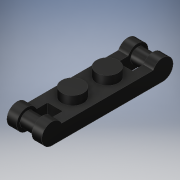
# Autodesk Inventor part: Weird circle things
Saved by Autodesk Inventor 2017 (Build 210142000, 142)
## iProperties
Created: 2018-05-11
Part Number: Weird circle things
Material: ABS Plastic
Document SubType Name: Modeling
Designer: Kyle
Density: 1.06 g/cm^3
Appearance: Glossy - Black
Author: Kyle
Autodesk Inventor part; units mm, degrees
ref_plane "YZ Plane" through (0, 0, 0) normal (1, 0, 0) x (0, 1, 0)
ref_plane "XZ Plane" through (0, 0, 0) normal (0, 1, 0) x (-1, 0, 0)
ref_plane "XY Plane" through (0, 0, 0) normal (0, 0, 1) x (1, 0, 0)
sketch "Sketch1" plane through (0, 0, 0) normal (0, 1, 0) x (-1, 0, 0)
  line L0 (0, 0) -> (7.7978, 0) construction
  line L1 (7.7978, 0) -> (7.7978, -21.1531) construction
  line L2 (7.7978, -21.1531) -> (0, -21.1531) construction
  line L3 (0, -21.1531) -> (0, 0) construction
  line L4 (7.7978, -10.5766) -> (7.7978, -2.7788) construction
  line L5 (7.7978, -2.7788) -> (0, -2.7788) construction
  line L6 (0, -2.7788) -> (0, -18.3744) construction
  line L7 (0, -18.3744) -> (7.7978, -18.3744) construction
  line L8 (7.7978, -18.3744) -> (7.7978, -2.7788) construction
  line L9 (7.7978, 0) -> (5.5905, 0) construction
  line L10 (5.5905, 0) -> (5.5905, -2.7788) construction
  line L11 (5.5905, -2.7788) -> (7.7978, -2.7788) construction
  line L12 (7.7978, -2.7788) -> (7.7978, 0) construction
  line L13 (7.7978, -10.5766) -> (0, -10.5766) construction
  line L14 (5.5905, -21.1531) -> (5.5905, -18.3744) construction
  line L15 (3.8989, 0) -> (3.8989, -21.1531) construction
  line L16 (2.2073, 0) -> (2.2073, -2.7788) construction
  line L17 (2.2073, -21.1531) -> (2.2073, -18.3744) construction
  line L18 (7.7978, 0) -> (7.7978, -21.1531)
  line L19 (7.7978, -21.1531) -> (5.5905, -21.1531)
  line L20 (5.5905, -21.1531) -> (5.5905, -18.3744)
  line L21 (5.5905, -18.3744) -> (2.2073, -18.3744)
  line L22 (2.2073, -18.3744) -> (2.2073, -21.1531)
  line L23 (2.2073, -21.1531) -> (0, -21.1531)
  line L24 (0, -21.1531) -> (0, 0)
  line L25 (0, 0) -> (2.2073, 0)
  line L26 (2.2073, 0) -> (2.2073, -2.7788)
  line L27 (2.2073, -2.7788) -> (5.5905, -2.7788)
  line L28 (5.5905, -2.7788) -> (5.5905, 0)
  line L29 (5.5905, 0) -> (7.7978, 0)
  dimension "d0" = 7.7978
  dimension "d1" = 21.1531
  dimension "d2" = 7.7978
  dimension "d3" = 7.7978
  dimension "d4" = 15.5956
  dimension "d5" = 2.2073
  constraints: 60 end point, 6 collinear, 6 parallel, 6 symmetric about line, 5 perpendicular, 4 midpoint, 3 horizontal, 2 point on line
  measures "d0" distance of L1.end L2.end
  measures "d1" distance of L0.end L1.end
  measures "d2" distance of L4.start L4.end
  measures "d3" distance of L7.end L6.end
  measures "d4" distance of L6.end L5.end
  measures "d5" distance of L11.end L10.end
extrude "Extrusion1" add sketch "Sketch1" along normal blind 3.236
sketch "Sketch2" plane through (0, 3.236, 0) normal (0, 1, 0) x (1, 0, 0)
  line L0 (0, 0) -> (0, 21.1531) construction
  line L1 (0, 10.5766) -> (-7.7978, 10.5766) construction
  line L2 (-7.7978, 21.1531) -> (-7.7978, 0) construction
  line L3 (0, 10.5766) -> (-3.8989, 10.5766) construction
  line L4 (-3.8989, 10.5766) -> (-3.8989, 6.6777) construction
  line L5 (-3.8989, 6.6777) -> (0, 6.6777) construction
  line L6 (0, 6.6777) -> (0, 10.5766) construction
  circle A0 centre (-3.8989, 6.6777) radius 2.4498
  dimension "d8" = 3.8989
  dimension "d9" = 3.8989
  dimension "d10" = 4.8997
  constraints: 10 end point, 2 midpoint, 2 parallel, 1 centre point, 1 coincident, 1 horizontal, 1 perpendicular
  measures "d8" distance of L5.end L4.end
  measures "d9" distance of L4.end L3.end
  measures "d10" diameter of A0
extrude "Extrusion2" add sketch "Sketch2" along normal blind 1.9837
pattern_linear "Rectangular Pattern1" count 2 spacing 7.7978 along (0, 0, -1) of "Extrusion2"
shell "Shell1" thickness 1.4732 removed faces 1 at (-3.335, 0, -7.9773)
sketch "Sketch3" plane through (-6.3246, 1.7628, -16.9012) normal (0, -1, 0) x (1, 0, 0)
  circle A0 centre (2.4257, 10.2235) radius 2.4498 construction
  circle A1 centre (2.4257, 2.4257) radius 2.4498 construction
  line L0 (2.4257, 10.2235) -> (2.4257, 2.4257) construction
  circle A2 centre (2.4257, 6.3246) radius 1.4491
  point P0 (6.3246, 16.9012)
  constraints: 2 end point, 1 centre point, 1 midpoint, 1 vertical
extrude "Extrusion3" add sketch "Sketch3" along normal up to surface (1.7628 mm away)
ref_plane "Work Plane1" through (0, 2.3178, 0) normal (0, -1, 0) x (1, 0, 0)
sketch "Sketch5" plane through (0, 2.3178, 0) normal (0, -1, 0) x (1, 0, 0)
  line L0 (-7.7978, -21.1531) -> (-7.7978, 0) construction
  line L1 (-7.7978, 0) -> (-7.7978, 1.8186) construction
  line L2 (-7.7978, 0) -> (-5.9792, 0) construction
  line L3 (-7.7978, 1.8186) -> (0, 1.8186) construction
  line L4 (0, 1.8186) -> (0, 4.1377) construction
  line L5 (0, 4.1377) -> (-7.7978, 4.1377) construction
  line L6 (-7.7978, 4.1377) -> (-7.7978, 1.8186) construction
  line L7 (-7.7978, 4.1377) -> (-5.5905, 4.1377) construction
  line L8 (-7.7978, 4.1377) -> (-5.5905, 4.1377) construction
  line L9 (-5.5905, 4.1377) -> (-2.2073, 4.1377) construction
  line L10 (-2.2073, 4.1377) -> (-2.2073, 3.4366) construction
  line L11 (-2.2073, 3.4366) -> (-5.5905, 3.4366) construction
  line L12 (-5.5905, 3.4366) -> (-5.5905, 4.1377) construction
  line L13 (-7.7978, 1.8186) -> (0, 1.8186)
  line L14 (0, 1.8186) -> (0, 4.1377)
  line L15 (0, 4.1377) -> (-2.2073, 4.1377)
  line L16 (-2.2073, 4.1377) -> (-2.2073, 3.4366)
  line L17 (-2.2073, 3.4366) -> (-5.5905, 3.4366)
  line L18 (-5.5905, 3.4366) -> (-5.5905, 4.1377)
  line L19 (-5.5905, 4.1377) -> (-7.7978, 4.1377)
  line L20 (-7.7978, 4.1377) -> (-7.7978, 1.8186)
  dimension "d28" = 1.8186
  dimension "d29" = 90
  dimension "d30" = 7.7978
  dimension "d31" = 2.319
  dimension "d32" = 2.2073
  dimension "d33" = 0
  dimension "d34" = 3.3833
  dimension "d35" = 0.701
  constraints: 40 end point, 6 perpendicular, 5 horizontal, 4 collinear, 4 parallel, 2 equal length, 1 vertical
  measures "d28" distance of L0.end L1.end
  measures "d29" angle of L2 L1
  measures "d30" distance of L5.end L4.end
  measures "d31" distance of L4.end L3.end
  measures "d32" distance of L5.end L7.end
  measures "d33" distance between parallel lines of L7 L8
  measures "d34" distance of L10.end L11.end
  measures "d35" distance of L9.end L10.end
revolve "Revolution1" add sketch "Sketch5" angle 360 about axis through (-7.7978, 2.3178, 1.8186) along (1, 0, 0)
sketch "Sketch6" plane through (-2.2073, 0, 0) normal (0, 0, 1) x (1, 0, 0)
  line L0 (2.2073, 0) -> (0, 0) projected
  line L1 (0, 0) -> (0, 3.236) projected
  line L2 (2.2073, 0) -> (0, 0)
  line L3 (0, 0) -> (0, 3.236)
  line L4 (0, 3.236) -> (2.2073, 3.236)
  line L5 (2.2073, 3.236) -> (2.2073, 0)
  line L6 (-3.3833, 0) -> (-5.5905, 0) projected
  line L7 (-3.3833, 0) -> (-3.3833, 3.236) projected
  line L8 (-5.5905, 0) -> (-3.3833, 0)
  line L9 (-3.3833, 0) -> (-3.3833, 3.236)
  line L10 (-3.3833, 3.236) -> (-5.5905, 3.236)
  line L11 (-5.5905, 3.236) -> (-5.5905, 0)
  constraints: 16 end point, 4 parallel, 2 horizontal, 2 perpendicular
extrude "Extrusion4" add sketch "Sketch6" along normal up to surface round surface about axis through (-1.1036, 2.3178, 1.8186) along (1, 0, 0) radius 2.319 far side no
ref_plane "Work Plane2" through (-5.5905, 0, -10.5766) normal (0, 0, 1) x (1, 0, 0)
mirror "Mirror1" about plane through (-5.5905, 0, -10.5766) normal (0, 0, 1) of "Revolution1", "Extrusion4"
body "Solid1"
